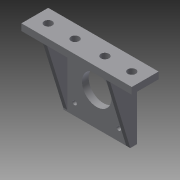
# Autodesk Inventor part: z motor mount
Saved by Autodesk Inventor 2014 SP1 (Build 180222100, 222)
## iProperties
Created: 2014-10-09
Part Number: z motor mount
Material: ABS Plastic
Document SubType Name: Modeling
Designer: Mon
Density: 1.06 g/cm^3
Appearance: Smooth - White
Author: Mon
Autodesk Inventor part; units mm, degrees
ref_plane "YZ Plane" through (0, 0, 0) normal (1, 0, 0) x (0, 1, 0)
ref_plane "XZ Plane" through (0, 0, 0) normal (0, 1, 0) x (-1, 0, 0)
ref_plane "XY Plane" through (0, 0, 0) normal (0, 0, 1) x (1, 0, 0)
sketch "Sketch1" plane through (0, 0, 0) normal (0, 0, 1) x (1, 0, 0)
  line L0 (0, 0) -> (82.3, 0)
  line L1 (82.3, 0) -> (82.3, 20)
  line L2 (82.3, 20) -> (0, 20)
  line L3 (0, 20) -> (0, 0)
  line L4 (-2.8173, 10) -> (83.4818, 10)
  line L5 (41.15, 24.9256) -> (41.15, -5.5134)
  line L6 (41.15, -5.5134) -> (20, -5.5134) construction
  line L7 (41.15, -5.5134) -> (62.3, -5.5134) construction
  line L8 (20, -5.5134) -> (20, 27.3565) construction
  line L9 (62.3, -5.5134) -> (62.3, 27.7135) construction
  line L10 (20, -5.5134) -> (10, -5.5134) construction
  line L11 (10, -5.5134) -> (10, 28.7251)
  circle A0 centre (10, 10) radius 3
  line L12 (20, -5.5134) -> (30, -5.5134) construction
  line L13 (30, -5.5134) -> (30, 27.7135)
  circle A1 centre (30, 10) radius 3
  line L14 (62.3, -5.5134) -> (72.3, -5.5134) construction
  line L15 (72.3, -5.5134) -> (72.3, 24.2533)
  line L16 (62.3, -5.5134) -> (52.3, -5.5134)
  line L17 (52.3, -5.5134) -> (52.3, 29.0456)
  circle A2 centre (52.3, 10) radius 3
  circle A3 centre (72.3, 10) radius 3
  dimension "d0" = 82.3
  dimension "d1" = 20
  dimension "d2" = 21.15
  dimension "d3" = 21.15
  dimension "d4" = 10
  dimension "d5" = 6
  dimension "d6" = 10
  dimension "d7" = 6
  dimension "d8" = 10
  dimension "d9" = 10
  dimension "d10" = 6
  dimension "d11" = 6
  constraints: 36 end point, 11 perpendicular, 10 point on line, 4 centre point, 3 parallel, 1 collinear, 1 horizontal
  measures "d0" distance of L2.end L1.end
  measures "d1" distance of L1.end L0.end
  measures "d2" distance of L5.end L6.end
  measures "d3" distance of L5.end L7.end
  measures "d4" distance of L6.end L10.end
  measures "d5" diameter of A0
  measures "d6" distance of L6.end L12.end
  measures "d7" diameter of A1
  measures "d8" distance of L7.end L14.end
  measures "d9" distance of L7.end L16.end
  measures "d10" diameter of A2
  measures "d11" diameter of A3
extrude "Extrusion1" add sketch "Sketch1" along normal blind 5 contours L3 L4 A0 L11 L0 | L11 A0 L4 A1 L13 L0 | L3 L2 L11 A0 L4 | L13 A1 L4 L5 L0 | L5 L4 A2 L17 L0 | A0 L11 L2 L13 A1 L4 | L17 A2 L4 A3 L15 L0 | L5 L2 L17 A2 L4 | L4 A1 L13 L2 L5 | L15 A3 L4 L1 L0 | A2 L17 L2 L15 A3 L4 | L4 A3 L15 L2 L1
sketch "Sketch2" plane through (0, 20, 0) normal (0, 1, 0) x (1, 0, 0)
  line L0 (82.3, 0) -> (0, 0) projected
  line L1 (0, 0) -> (0, -5) projected
  line L2 (82.3, 0) -> (82.3, -5) projected
  line L3 (41.15, 64.2436) -> (41.15, -26.8176)
  line L4 (41.15, 0) -> (66.15, 0)
  line L5 (66.15, 0) -> (66.15, 50)
  line L6 (66.15, 50) -> (16.15, 50)
  line L7 (16.15, 50) -> (16.15, 0)
  circle A0 centre (41.15, 25) radius 11
  line L8 (41.15, 64.2436) -> (57.65, 64.2436)
  line L9 (57.65, 6.1421) -> (5.0097, 6.1421)
  circle A1 centre (57.65, 41.5) radius 1.6
  circle A2 centre (24.65, 41.5) radius 1.6
  circle A3 centre (24.65, 10.5) radius 1.6
  circle A4 centre (57.65, 10.5) radius 1.6
  dimension "d14" = 25
  dimension "d15" = 50
  dimension "d16" = 50
  dimension "d17" = 22
  dimension "d20" = 16.5
  dimension "d22" = 3.2
  dimension "d23" = 3.2
  dimension "d24" = 3.2
  dimension "d25" = 3.2
  constraints: 14 end point, 5 centre point, 4 point on line, 3 parallel, 2 perpendicular, 1 midpoint
  measures "d14" distance of L4.start L4.end
  measures "d15" distance of L4.end L5.end
  measures "d16" distance of L5.end L6.end
  measures "d17" diameter of A0
  measures "d20" distance of L3.start L8.end
  measures "d22" diameter of A1
  measures "d23" diameter of A2
  measures "d24" diameter of A3
  measures "d25" diameter of A4
extrude "Extrusion2" add sketch "Sketch2" against normal blind 5 contours L0 L3 A0 L6 L5 | L0 L7 L9 L3 | L9 L7 L6 L3 A0
sketch "Sketch3" plane through (16.15, 20, -50) normal (-1, 0, 0) x (0, 0, 1)
  line L0 (50, -5) -> (0, -5) projected
  line L1 (50, 0) -> (50, -5) projected
  line L2 (1.2041, -5) -> (50, -20)
  line L3 (50, -20) -> (50, -5)
  line L4 (50, -20) -> (50, -5)
  line L5 (50, -5) -> (1.2041, -5)
  constraints: 8 end point, 2 collinear, 1 perpendicular, 1 point on line
extrude "Extrusion3" add sketch "Sketch3" against normal blind 3
sketch "Sketch4" plane through (66.15, 20, 0) normal (1, 0, 0) x (0, 0, -1)
  line L0 (50, -5) -> (0, -5) projected
  line L1 (0, -20) -> (50, -5)
  line L2 (50, -5) -> (1.261, -5)
  line L3 (0, -5) -> (0, -20)
  constraints: 6 end point, 1 coincident, 1 perpendicular, 1 point on line
extrude "Extrusion4" add sketch "Sketch4" against normal blind 3
body "Solid1"
